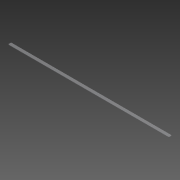
# Autodesk Inventor part: bottom
Saved by Autodesk Inventor 2013 (Build 170138000, 138)
## iProperties
Created: 2013-04-25
Part Number: bottom
Material: Polycarbonate, Clear
Document SubType Name: Sheet Metal
Designer: Chris
Density: 1 g/cm^3
Sheet Metal Rule: Default
Author: Chris
Autodesk Inventor part; units mm, degrees
ref_plane "YZ Plane" through (0, 0, 0) normal (1, 0, 0) x (0, 1, 0)
ref_plane "XZ Plane" through (0, 0, 0) normal (0, 1, 0) x (-1, 0, 0)
ref_plane "XY Plane" through (0, 0, 0) normal (0, 0, 1) x (1, 0, 0)
sketch "Sketch1" plane through (0, 0, 0) normal (0, 1, 0) x (-1, 0, 0)
  line L0 (6.096, 0) -> (1340.104, 0)
  line L1 (1346.2, 6.096) -> (1346.2, 19.304)
  line L2 (1340.104, 25.4) -> (6.096, 25.4)
  line L3 (0, 19.304) -> (0, 6.096)
  arc A0 (6.096, 25.4) -> (0, 19.304) centre (6.096, 19.304) ccw
  arc A1 (0, 6.096) -> (6.096, 0) centre (6.096, 6.096) ccw
  arc A2 (1340.104, 0) -> (1346.2, 6.096) centre (1340.104, 6.096) ccw
  arc A3 (1346.2, 19.304) -> (1340.104, 25.4) centre (1340.104, 19.304) ccw
  point P0 (0, 0)
  point P1 (1346.2, 25.4)
  point P2 (1346.2, 0)
  point P3 (0, 25.4)
  dimension "d0" = 1346.2
  dimension "d1" = 25.4
  dimension "d2" = 6.096
  measures "d0" distance of point (0, 25.4) point (1346.2, 25.4)
  measures "d1" distance of point (1346.2, 25.4) point (1346.2, 0)
  measures "d2" radius of A0
extrude "Plate1" add sketch "Sketch1" along normal blind 3.048
equation "\"BendRadius\" = Thickness"
equation "\"BendReliefWidth\" = Thickness"
equation "\"BendReliefDepth\" = 0.5 * Thickness"
equation "\"CornerReliefSize\" = 4 * Thickness"
equation "\"MinimumRemnant\" = 2 * Thickness"
equation "\"TransitionRadius\" = BendRadius"
equation "\"JacobiRadiusSize\" = BendRadius"
equation "\"GapSize\" = Thickness"
equation "\"d3\" = BendRadius"
equation "\"Thickness\" = 3.048"
body "Solid1"
